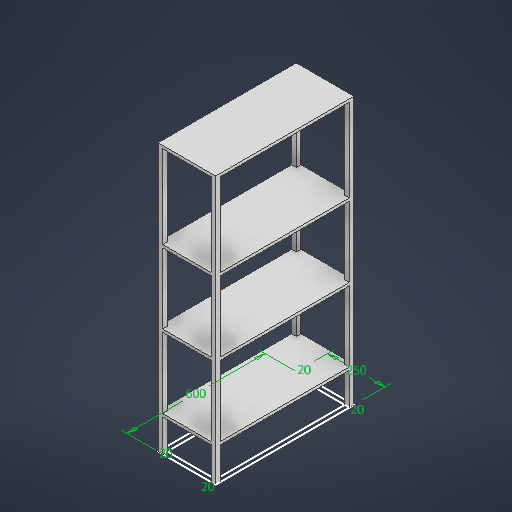
# Autodesk Inventor part: Pieza2
Saved by Autodesk Inventor 2026 (Build 300175050, 175E)
## iProperties
Created: 2025-07-24
Part Number: Pieza2
Material: Genérico
Document SubType Name: Modeling
Designer: diazg
Density: 1 g/cm^3
Appearance: Valor por defecto
Author: diazg
Autodesk Inventor part; units mm, degrees
ref_plane "YZ Plane" through (0, 0, 0) normal (1, 0, 0) x (0, 1, 0)
ref_plane "XZ Plane" through (0, 0, 0) normal (0, 1, 0) x (-1, 0, 0)
ref_plane "XY Plane" through (0, 0, 0) normal (0, 0, 1) x (1, 0, 0)
sketch "Boceto1" plane through (0, 0, 0) normal (0, 1, 0) x (-1, 0, 0)
  line L0 (0, 0) -> (250, 0)
  line L1 (250, 0) -> (250, -600)
  line L2 (250, -600) -> (0, -600)
  line L3 (0, -600) -> (0, 0)
  line L4 (250, 0) -> (250, -20)
  line L5 (250, -20) -> (0, -20)
  line L6 (0, 0) -> (20, 0)
  line L7 (20, 0) -> (20, -600)
  line L8 (0, -600) -> (0, -580)
  line L9 (0, -580) -> (250, -580)
  line L10 (250, -600) -> (230, -600)
  line L11 (230, -600) -> (230, 0)
  point P0 (20, -20)
  point P1 (20, -580)
  point P2 (230, -580)
  point P3 (230, -20)
  dimension "d0" = 250
  dimension "d1" = 600
  dimension "d2" = 20
  dimension "d3" = 20
  dimension "d4" = 20
  dimension "d5" = 20
  constraints: 24 end point, 8 point on line, 5 perpendicular, 2 parallel, 1 horizontal
  measures "d0" distance of L1.end L2.end
  measures "d1" distance of L0.end L1.end
  measures "d2" distance of L0.end L4.end
  measures "d3" distance of L0.start L6.end
  measures "d4" distance of L2.end L8.end
  measures "d5" distance of L1.end L10.end
extrude "Extrusión1" add sketch "Boceto1" along normal blind 1160 contours L0 L7 L5 L3 | L0 L1 L5 L11 | L9 L7 L2 L3 | L9 L1 L2 L11
extrude "Extrusión2" add sketch "Boceto1" along normal blind 1160 contours L0 L11 L5 L7 | L5 L7 L9 L3 | L5 L11 L9 L7 | L5 L1 L9 L11 | L9 L11 L2 L7
extrude "Extrusión3" cut sketch "Boceto1" along normal blind 1147.5 contours L0 L11 L5 L7 | L5 L7 L9 L3 | L5 L11 L9 L7 | L5 L1 L9 L11 | L9 L11 L2 L7
extrude "Extrusión4" add sketch "Boceto1" along normal blind 787.5 contours L0 L11 L5 L7 | L5 L7 L9 L3 | L5 L11 L9 L7 | L5 L1 L9 L11 | L9 L11 L2 L7
extrude "Extrusión5" cut sketch "Boceto1" along normal blind 775 contours L0 L11 L5 L7 | L5 L7 L9 L3 | L5 L11 L9 L7 | L5 L1 L9 L11 | L9 L11 L2 L7
extrude "Extrusión6" add sketch "Boceto1" along normal blind 470 contours L0 L11 L5 L7 | L5 L7 L9 L3 | L5 L11 L9 L7 | L5 L1 L9 L11 | L9 L11 L2 L7
extrude "Extrusión7" cut sketch "Boceto1" along normal blind 457.5 contours L0 L11 L5 L7 | L5 L7 L9 L3 | L5 L11 L9 L7 | L5 L1 L9 L11 | L9 L11 L2 L7
extrude "Extrusión8" add sketch "Boceto1" along normal blind 152.5 contours L0 L11 L5 L7 | L5 L7 L9 L3 | L5 L11 L9 L7 | L5 L1 L9 L11 | L9 L11 L2 L7
extrude "Extrusión9" cut sketch "Boceto1" along normal blind 140 contours L0 L11 L5 L7 | L5 L7 L9 L3 | L5 L11 L9 L7 | L5 L1 L9 L11 | L9 L11 L2 L7
